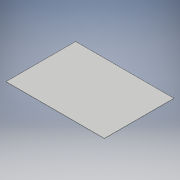
# Autodesk Inventor part: liaison
Saved by Autodesk Inventor 2017 (Build 210142000, 142)
## iProperties
Created: 2017-03-09
Part Number: liaison
Material: Generic
Document SubType Name: Modeling
Designer: LaFaucheuse
Density: 1 g/cm^3
Appearance: Default
Author: LaFaucheuse
Autodesk Inventor part; units mm, degrees
ref_plane "YZ Plane" through (0, 0, 0) normal (1, 0, 0) x (0, 1, 0)
ref_plane "XZ Plane" through (0, 0, 0) normal (0, 1, 0) x (-1, 0, 0)
ref_plane "XY Plane" through (0, 0, 0) normal (0, 0, 1) x (1, 0, 0)
sketch "Esquisse1" plane through (0, 0, 0) normal (0, 1, 0) x (-1, 0, 0)
  line L0 (0, 0) -> (297, 0)
  line L1 (297, 0) -> (297, -210)
  line L2 (297, -210) -> (0, -210)
  line L3 (0, -210) -> (0, 0)
  dimension "d3" = 297
  dimension "d4" = 210
  constraints: 8 end point, 2 parallel, 1 horizontal, 1 perpendicular
  measures "d3" distance of L1.end L2.end
  measures "d4" distance of L0.end L1.end
extrude "Extrusion1" add sketch "Esquisse1" along normal blind 0.5
